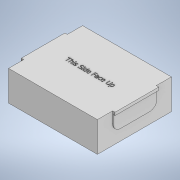
# Autodesk Inventor part: iRobot_filter
Saved by Autodesk Inventor 2020 (Build 240168000, 168)
## iProperties
Created: 2020-04-05
Part Number: iRobot_filter
Material: Generic
Document SubType Name: Modeling
Designer: Clevo
Density: 1 g/cm^3
Appearance: Default
Author: Clevo
Autodesk Inventor part; units mm, degrees
ref_plane "YZ Plane" through (0, 0, 0) normal (1, 0, 0) x (0, 1, 0)
ref_plane "XZ Plane" through (0, 0, 0) normal (0, 1, 0) x (-1, 0, 0)
ref_plane "XY Plane" through (0, 0, 0) normal (0, 0, 1) x (1, 0, 0)
sketch "Sketch1" plane through (0, 0, 0) normal (0, 1, 0) x (-1, 0, 0)
  line L0 (-30.48, -25.4) -> (30.48, -25.4)
  line L1 (30.48, -25.4) -> (30.48, 25.4)
  line L2 (30.48, 25.4) -> (-30.48, 25.4)
  line L3 (-30.48, 25.4) -> (-30.48, -25.4)
  line L4 (-30.48, -25.4) -> (30.48, 25.4) construction
  line L5 (30.48, -25.4) -> (-30.48, 25.4) construction
  point P0 (0, 0)
  dimension "d0" = 50.8
  dimension "d1" = 60.96
  constraints: 12 end point, 2 midpoint, 2 parallel, 1 horizontal, 1 perpendicular
  measures "d0" distance of L0.end L1.end
  measures "d1" distance of L1.end L2.end
extrude "Extrusion1" add sketch "Sketch1" along normal blind 20.6629
sketch "Sketch2" plane through (30.48, 0, 25.4) normal (1, 0, 0) x (0, 0, -1)
  line L0 (0, 0) -> (50.8, 0) projected
  line L1 (50.8, 0) -> (50.8, 20.6629) projected
  line L2 (0, 20.6629) -> (50.8, 20.6629) projected
  line L3 (0, 0) -> (0, 20.6629) projected
  line L4 (0, 20.6629) -> (50.8, 20.6629) projected
  line L5 (10.4, 20.6629) -> (40.4, 20.6629)
  line L6 (40.4, 20.6629) -> (40.4, 7.9629)
  line L7 (40.4, 7.9629) -> (10.4, 7.9629)
  line L8 (10.4, 7.9629) -> (10.4, 20.6629)
  point P0 (25.4, 0)
  point P1 (25.4, 20.6629)
  point P2 (25.4, 20.6629)
  point P3 (10.4, 20.6629)
  dimension "d4" = 12.7
  dimension "d5" = 30
  constraints: 8 end point, 2 midpoint, 2 parallel, 1 coincident, 1 horizontal, 1 perpendicular, 1 point on line
  measures "d4" distance of L5.end L6.end
  measures "d5" distance of L6.end L7.end
extrude "Extrusion2" add sketch "Sketch2" along normal blind 0.5 contours L2 L6 L7 L8
fillet "Fillet1" radius 5 2 edges at (30.73, 7.9629, 15) (30.73, 7.9629, -15)
sketch "Sketch3" plane through (30.98, 0, 25.4) normal (1, 0, 0) x (0, 0, -1)
  arc A0 (35.4, 7.9629) -> (40.4, 12.9629) centre (35.4, 12.9629) ccw projected
  line L0 (40.4, 12.9629) -> (40.4, 20.6629) projected
  line L1 (40.4, 20.6629) -> (10.4, 20.6629) projected
  line L2 (10.4, 20.6629) -> (10.4, 12.9629) projected
  arc A1 (10.4, 12.9629) -> (15.4, 7.9629) centre (15.4, 12.9629) ccw projected
  line L3 (15.4, 7.9629) -> (35.4, 7.9629) projected
  line L4 (40.4, 20.6629) -> (10.4, 20.6629) projected
  line L5 (40.4, 12.9629) -> (40.4, 20.6629) projected
  line L6 (10.4, 20.6629) -> (40.4, 20.6629)
  line L7 (40.4, 20.6629) -> (40.4, 18.6629)
  line L8 (40.4, 18.6629) -> (10.4, 18.6629)
  line L9 (10.4, 18.6629) -> (10.4, 20.6629)
  point P0 (25.4, 0)
  point P1 (10.4, 18.6629)
  dimension "d9" = 2
  constraints: 8 end point, 2 parallel, 1 horizontal, 1 perpendicular, 1 point on line
  measures "d9" distance between parallel lines of L1 L8
extrude "Extrusion3" add sketch "Sketch3" along normal blind 1.17 contours L8 L2 L1 L0
mirror "Mirror1" about plane through (0, 0, 0) normal (1, 0, 0) of "Extrusion2", "Fillet1", "Extrusion3"
sketch "Sketch4" plane through (0, 20.6629, 0) normal (0, 1, 0) x (1, 0, 0)
  line L0 (-16.5843, 2.036) -> (16.3633, 2.036) construction
  line L1 (16.3633, 2.036) -> (16.3633, -1.9901) construction
  line L2 (16.3633, -1.9901) -> (-16.5843, -1.9901) construction
  line L3 (-16.5843, -1.9901) -> (-16.5843, 2.036) construction
  line L4 (-15.5642, -1.1479) -> (-15.5642, 1.5395)
  line L5 (-15.5642, 1.5395) -> (-16.5867, 1.5395)
  line L6 (-16.5867, 1.5395) -> (-16.5867, 1.9001)
  line L7 (-16.5867, 1.9001) -> (-14.1365, 1.9001)
  line L8 (-14.1365, 1.9001) -> (-14.1365, 1.5395)
  line L9 (-14.1365, 1.5395) -> (-15.1591, 1.5395)
  line L10 (-15.1591, 1.5395) -> (-15.1591, -1.1479)
  line L11 (-15.1591, -1.1479) -> (-15.5642, -1.1479)
  line L12 (-12.0617, -1.1479) -> (-12.447, -1.1479)
  line L13 (-12.447, -1.1479) -> (-12.447, 0.1563)
  spline S0 degree 2 poles (-12.447, 0.1563) (-12.447, 0.3144) (-12.4766, 0.5861) (-12.5211, 0.6676) knots 0 0 0 1 2 2 2
  spline S1 degree 2 poles (-12.5211, 0.6676) (-12.568, 0.7541) (-12.736, 0.838) (-12.8792, 0.838) knots 0 0 0 1 2 2 2
  spline S2 degree 2 poles (-12.8792, 0.838) (-13.0225, 0.838) (-13.3263, 0.6849) (-13.472, 0.5614) knots 0 0 0 1 2 2 2
  line L14 (-13.472, 0.5614) -> (-13.472, -1.1479)
  line L15 (-13.472, -1.1479) -> (-13.8574, -1.1479)
  line L16 (-13.8574, -1.1479) -> (-13.8574, 2.036)
  line L17 (-13.8574, 2.036) -> (-13.472, 2.036)
  line L18 (-13.472, 2.036) -> (-13.472, 0.885)
  spline S3 degree 2 poles (-13.472, 0.885) (-13.2991, 1.0406) (-12.9657, 1.2036) (-12.778, 1.2036) knots 0 0 0 1 2 2 2
  spline S4 degree 2 poles (-12.778, 1.2036) (-12.4421, 1.2036) (-12.0617, 0.759) (-12.0617, 0.3366) knots 0 0 0 1 2 2 2
  line L19 (-12.0617, 0.3366) -> (-12.0617, -1.1479)
  line L20 (-11.128, -1.1479) -> (-11.5133, -1.1479)
  line L21 (-11.5133, -1.1479) -> (-11.5133, 1.1394)
  line L22 (-11.5133, 1.1394) -> (-11.128, 1.1394)
  line L23 (-11.128, 1.1394) -> (-11.128, -1.1479)
  line L24 (-11.1008, 1.5198) -> (-11.538, 1.5198)
  line L25 (-11.538, 1.5198) -> (-11.538, 1.9199)
  line L26 (-11.538, 1.9199) -> (-11.1008, 1.9199)
  line L27 (-11.1008, 1.9199) -> (-11.1008, 1.5198)
  spline S5 degree 2 poles (-9.9449, -1.2022) (-10.1746, -1.2022) (-10.5722, -1.0787) (-10.7032, -1.0095) knots 0 0 0 1 2 2 2
  line L28 (-10.7032, -1.0095) -> (-10.7032, -0.5773)
  line L29 (-10.7032, -0.5773) -> (-10.6834, -0.5773)
  spline S6 degree 2 poles (-10.6834, -0.5773) (-10.634, -0.6168) (-10.5006, -0.7107) (-10.3895, -0.7625) knots 0 0 0 1 2 2 2
  spline S7 degree 2 poles (-10.3895, -0.7625) (-10.2931, -0.8095) (-10.056, -0.8786) (-9.93, -0.8786) knots 0 0 0 1 2 2 2
  spline S8 degree 2 poles (-9.93, -0.8786) (-9.8387, -0.8786) (-9.6287, -0.8366) (-9.5793, -0.8021) knots 0 0 0 1 2 2 2
  spline S9 degree 2 poles (-9.5793, -0.8021) (-9.5077, -0.7551) (-9.4435, -0.6489) (-9.4435, -0.5402) knots 0 0 0 1 2 2 2
  spline S10 degree 2 poles (-9.4435, -0.5402) (-9.4435, -0.4044) (-9.5917, -0.2636) (-9.7818, -0.2167) knots 0 0 0 1 2 2 2
  spline S11 degree 2 poles (-9.7818, -0.2167) (-9.8559, -0.1994) (-10.0931, -0.15) (-10.1943, -0.1228) knots 0 0 0 1 2 2 2
  spline S12 degree 2 poles (-10.1943, -0.1228) (-10.4562, -0.0462) (-10.6933, 0.2699) (-10.6933, 0.4947) knots 0 0 0 1 2 2 2
  spline S13 degree 2 poles (-10.6933, 0.4947) (-10.6933, 0.8059) (-10.2264, 1.1937) (-9.8411, 1.1937) knots 0 0 0 1 2 2 2
  spline S14 degree 2 poles (-9.8411, 1.1937) (-9.6509, 1.1937) (-9.2656, 1.0999) (-9.1347, 1.0282) knots 0 0 0 1 2 2 2
  line L30 (-9.1347, 1.0282) -> (-9.1347, 0.6157)
  line L31 (-9.1347, 0.6157) -> (-9.1545, 0.6157)
  spline S15 degree 2 poles (-9.1545, 0.6157) (-9.3027, 0.7343) (-9.6633, 0.8701) (-9.8485, 0.8701) knots 0 0 0 1 2 2 2
  spline S16 degree 2 poles (-9.8485, 0.8701) (-10.0387, 0.8701) (-10.3005, 0.7096) (-10.3005, 0.549) knots 0 0 0 1 2 2 2
  spline S17 degree 2 poles (-10.3005, 0.549) (-10.3005, 0.4033) (-10.1449, 0.2625) (-9.972, 0.2181) knots 0 0 0 1 2 2 2
  spline S18 degree 2 poles (-9.972, 0.2181) (-9.8881, 0.1958) (-9.6756, 0.1514) (-9.5595, 0.1242) knots 0 0 0 1 2 2 2
  spline S19 degree 2 poles (-9.5595, 0.1242) (-9.3076, 0.06) (-9.0507, -0.2339) (-9.0507, -0.4884) knots 0 0 0 1 2 2 2
  spline S20 degree 2 poles (-9.0507, -0.4884) (-9.0507, -0.6366) (-9.1668, -0.8984) (-9.2804, -0.9947) knots 0 0 0 1 2 2 2
  spline S21 degree 2 poles (-9.2804, -0.9947) (-9.4015, -1.096) (-9.7102, -1.2022) (-9.9449, -1.2022) knots 0 0 0 1 2 2 2
  spline S22 degree 2 poles (-6.5041, -1.2022) (-6.8351, -1.2022) (-7.2995, -1.0639) (-7.5045, -0.9651) knots 0 0 0 1 2 2 2
  line L32 (-7.5045, -0.9651) -> (-7.5045, -0.4563)
  line L33 (-7.5045, -0.4563) -> (-7.4748, -0.4563)
  spline S23 degree 2 poles (-7.4748, -0.4563) (-7.2748, -0.644) (-6.7684, -0.8515) (-6.5338, -0.8515) knots 0 0 0 1 2 2 2
  spline S24 degree 2 poles (-6.5338, -0.8515) (-6.1978, -0.8515) (-5.8545, -0.5723) (-5.8545, -0.3426) knots 0 0 0 1 2 2 2
  spline S25 degree 2 poles (-5.8545, -0.3426) (-5.8545, -0.1598) (-6.0348, 0.0674) (-6.23, 0.1242) knots 0 0 0 1 2 2 2
  spline S26 degree 2 poles (-6.23, 0.1242) (-6.3708, 0.1637) (-6.6054, 0.2181) (-6.7808, 0.2625) knots 0 0 0 1 2 2 2
  spline S27 degree 2 poles (-6.7808, 0.2625) (-6.9389, 0.3045) (-7.1883, 0.4305) (-7.2847, 0.5318) knots 0 0 0 1 2 2 2
  spline S28 degree 2 poles (-7.2847, 0.5318) (-7.3785, 0.633) (-7.4823, 0.9047) (-7.4823, 1.0826) knots 0 0 0 1 2 2 2
  spline S29 degree 2 poles (-7.4823, 1.0826) (-7.4823, 1.4531) (-6.9043, 1.9545) (-6.4572, 1.9545) knots 0 0 0 1 2 2 2
  spline S30 degree 2 poles (-6.4572, 1.9545) (-6.2003, 1.9545) (-5.7458, 1.8532) (-5.5507, 1.7569) knots 0 0 0 1 2 2 2
  line L34 (-5.5507, 1.7569) -> (-5.5507, 1.2728)
  line L35 (-5.5507, 1.2728) -> (-5.5803, 1.2728)
  spline S31 degree 2 poles (-5.5803, 1.2728) (-5.7261, 1.4061) (-6.1806, 1.6037) (-6.43, 1.6037) knots 0 0 0 1 2 2 2
  spline S32 degree 2 poles (-6.43, 1.6037) (-6.7116, 1.6037) (-7.0599, 1.3395) (-7.0599, 1.1246) knots 0 0 0 1 2 2 2
  spline S33 degree 2 poles (-7.0599, 1.1246) (-7.0599, 0.9319) (-6.8549, 0.7022) (-6.6622, 0.6503) knots 0 0 0 1 2 2 2
  spline S34 degree 2 poles (-6.6622, 0.6503) (-6.5338, 0.6157) (-6.1608, 0.5268) (-6.0373, 0.4898) knots 0 0 0 1 2 2 2
  spline S35 degree 2 poles (-6.0373, 0.4898) (-5.7236, 0.3934) (-5.4321, 0.0056) (-5.4321, -0.2784) knots 0 0 0 1 2 2 2
  spline S36 degree 2 poles (-5.4321, -0.2784) (-5.4321, -0.4587) (-5.5779, -0.8045) (-5.7088, -0.9256) knots 0 0 0 1 2 2 2
  spline S37 degree 2 poles (-5.7088, -0.9256) (-5.8545, -1.0589) (-6.225, -1.2022) (-6.5041, -1.2022) knots 0 0 0 1 2 2 2
  line L36 (-4.6566, -1.1479) -> (-5.0419, -1.1479)
  line L37 (-5.0419, -1.1479) -> (-5.0419, 1.1394)
  line L38 (-5.0419, 1.1394) -> (-4.6566, 1.1394)
  line L39 (-4.6566, 1.1394) -> (-4.6566, -1.1479)
  line L40 (-4.6294, 1.5198) -> (-5.0666, 1.5198)
  line L41 (-5.0666, 1.5198) -> (-5.0666, 1.9199)
  line L42 (-5.0666, 1.9199) -> (-4.6294, 1.9199)
  line L43 (-4.6294, 1.9199) -> (-4.6294, 1.5198)
  line L44 (-2.3323, -1.1479) -> (-2.7176, -1.1479)
  line L45 (-2.7176, -1.1479) -> (-2.7176, -0.9157)
  spline S38 degree 2 poles (-2.7176, -0.9157) (-2.8065, -0.9898) (-2.9374, -1.0886) (-3.0263, -1.1306) knots 0 0 0 1 2 2 2
  spline S39 degree 2 poles (-3.0263, -1.1306) (-3.1079, -1.1701) (-3.2832, -1.2121) (-3.3993, -1.2121) knots 0 0 0 1 2 2 2
  spline S40 degree 2 poles (-3.3993, -1.2121) (-3.587, -1.2121) (-3.9032, -1.0565) (-4.0144, -0.9058) knots 0 0 0 1 2 2 2
  spline S41 degree 2 poles (-4.0144, -0.9058) (-4.1255, -0.7551) (-4.249, -0.3105) (-4.249, -0.0215) knots 0 0 0 1 2 2 2
  spline S42 degree 2 poles (-4.249, -0.0215) (-4.249, 0.2798) (-4.0934, 0.7195) (-3.9575, 0.885) knots 0 0 0 1 2 2 2
  spline S43 degree 2 poles (-3.9575, 0.885) (-3.8316, 1.0332) (-3.4784, 1.2036) (-3.2832, 1.2036) knots 0 0 0 1 2 2 2
  spline S44 degree 2 poles (-3.2832, 1.2036) (-3.1128, 1.2036) (-2.8584, 1.127) (-2.7176, 1.048) knots 0 0 0 1 2 2 2
  line L46 (-2.7176, 1.048) -> (-2.7176, 2.036)
  line L47 (-2.7176, 2.036) -> (-2.3323, 2.036)
  line L48 (-2.3323, 2.036) -> (-2.3323, -1.1479)
  line L49 (-2.7176, -0.5921) -> (-2.7176, 0.7294)
  spline S45 degree 2 poles (-2.7176, 0.7294) (-2.8609, 0.7985) (-3.0881, 0.8504) (-3.219, 0.8504) knots 0 0 0 1 2 2 2
  spline S46 degree 2 poles (-3.219, 0.8504) (-3.5154, 0.8504) (-3.8513, 0.4058) (-3.8513, -0.0141) knots 0 0 0 1 2 2 2
  spline S47 degree 2 poles (-3.8513, -0.0141) (-3.8513, -0.4192) (-3.5945, -0.8465) (-3.3104, -0.8465) knots 0 0 0 1 2 2 2
  spline S48 degree 2 poles (-3.3104, -0.8465) (-3.1597, -0.8465) (-2.8534, -0.7082) (-2.7176, -0.5921) knots 0 0 0 1 2 2 2
  spline S49 degree 2 poles (-0.7811, -1.1997) (-1.3294, -1.1997) (-1.9321, -0.5847) (-1.9321, -0.0166) knots 0 0 0 1 2 2 2
  spline S50 degree 2 poles (-1.9321, -0.0166) (-1.9321, 0.5416) (-1.3467, 1.2036) (-0.875, 1.2036) knots 0 0 0 1 2 2 2
  spline S51 degree 2 poles (-0.875, 1.2036) (-0.6625, 1.2036) (-0.334, 1.0801) (-0.213, 0.9492) knots 0 0 0 1 2 2 2
  spline S52 degree 2 poles (-0.213, 0.9492) (-0.0895, 0.8183) (0.0414, 0.4404) (0.0414, 0.1662) knots 0 0 0 1 2 2 2
  line L50 (0.0414, 0.1662) -> (0.0414, -0.0438)
  line L51 (0.0414, -0.0438) -> (-1.5419, -0.0438)
  spline S53 degree 2 poles (-1.5419, -0.0438) (-1.5419, -0.4414) (-1.1417, -0.8638) (-0.786, -0.8638) knots 0 0 0 1 2 2 2
  spline S54 degree 2 poles (-0.786, -0.8638) (-0.6601, -0.8638) (-0.4155, -0.807) (-0.3167, -0.7625) knots 0 0 0 1 2 2 2
  spline S55 degree 2 poles (-0.3167, -0.7625) (-0.213, -0.7131) (-0.0697, -0.6267) (-0.0228, -0.5872) knots 0 0 0 1 2 2 2
  line L52 (-0.0228, -0.5872) -> (-0.0006, -0.5872)
  line L53 (-0.0006, -0.5872) -> (-0.0006, -1.0071)
  spline S56 degree 2 poles (-0.0006, -1.0071) (-0.0673, -1.0342) (-0.2698, -1.1133) (-0.3489, -1.1355) knots 0 0 0 1 2 2 2
  spline S57 degree 2 poles (-0.3489, -1.1355) (-0.46, -1.1676) (-0.6428, -1.1997) (-0.7811, -1.1997) knots 0 0 0 1 2 2 2
  spline S58 degree 2 poles (-0.334, 0.2502) (-0.339, 0.4058) (-0.4032, 0.633) (-0.4649, 0.7096) knots 0 0 0 1 2 2 2
  spline S59 degree 2 poles (-0.4649, 0.7096) (-0.5316, 0.796) (-0.7416, 0.8874) (-0.8972, 0.8874) knots 0 0 0 1 2 2 2
  spline S60 degree 2 poles (-0.8972, 0.8874) (-1.0503, 0.8874) (-1.2652, 0.796) (-1.3541, 0.7071) knots 0 0 0 1 2 2 2
  spline S61 degree 2 poles (-1.3541, 0.7071) (-1.4406, 0.6157) (-1.5295, 0.3959) (-1.5419, 0.2502) knots 0 0 0 1 2 2 2
  line L54 (-1.5419, 0.2502) -> (-0.334, 0.2502)
  line L55 (3.5933, 1.5395) -> (2.1755, 1.5395)
  line L56 (2.1755, 1.5395) -> (2.1755, 0.68)
  line L57 (2.1755, 0.68) -> (3.534, 0.68)
  line L58 (3.534, 0.68) -> (3.534, 0.3193)
  line L59 (3.534, 0.3193) -> (2.1755, 0.3193)
  line L60 (2.1755, 0.3193) -> (2.1755, -1.1479)
  line L61 (2.1755, -1.1479) -> (1.7704, -1.1479)
  line L62 (1.7704, -1.1479) -> (1.7704, 1.9001)
  line L63 (1.7704, 1.9001) -> (3.5933, 1.9001)
  line L64 (3.5933, 1.9001) -> (3.5933, 1.5395)
  spline S62 degree 2 poles (5.2013, -0.9058) (5.1543, -0.9404) (4.9963, -1.0639) (4.9222, -1.1009) knots 0 0 0 1 2 2 2
  spline S63 degree 2 poles (4.9222, -1.1009) (4.8209, -1.1553) (4.6307, -1.2121) (4.4578, -1.2121) knots 0 0 0 1 2 2 2
  spline S64 degree 2 poles (4.4578, -1.2121) (4.317, -1.2121) (4.0626, -1.1059) (3.9663, -1.0095) knots 0 0 0 1 2 2 2
  spline S65 degree 2 poles (3.9663, -1.0095) (3.8749, -0.9157) (3.7637, -0.639) (3.7637, -0.4859) knots 0 0 0 1 2 2 2
  spline S66 degree 2 poles (3.7637, -0.4859) (3.7637, -0.2488) (3.9638, 0.0872) (4.1812, 0.1835) knots 0 0 0 1 2 2 2
  spline S67 degree 2 poles (4.1812, 0.1835) (4.3738, 0.2724) (4.8975, 0.3391) (5.2013, 0.3564) knots 0 0 0 1 2 2 2
  line L65 (5.2013, 0.3564) -> (5.2013, 0.4305)
  spline S68 degree 2 poles (5.2013, 0.4305) (5.2013, 0.5639) (5.1198, 0.7294) (5.0457, 0.7763) knots 0 0 0 1 2 2 2
  spline S69 degree 2 poles (5.0457, 0.7763) (4.9716, 0.8232) (4.7591, 0.8529) (4.6455, 0.8529) knots 0 0 0 1 2 2 2
  spline S70 degree 2 poles (4.6455, 0.8529) (4.5121, 0.8529) (4.1515, 0.7738) (3.9712, 0.6972) knots 0 0 0 1 2 2 2
  line L66 (3.9712, 0.6972) -> (3.949, 0.6972)
  line L67 (3.949, 0.6972) -> (3.949, 1.09)
  spline S71 degree 2 poles (3.949, 1.09) (4.0552, 1.1196) (4.4529, 1.1937) (4.648, 1.1937) knots 0 0 0 1 2 2 2
  spline S72 degree 2 poles (4.648, 1.1937) (4.8851, 1.1937) (5.2087, 1.1196) (5.3371, 1.0233) knots 0 0 0 1 2 2 2
  spline S73 degree 2 poles (5.3371, 1.0233) (5.4631, 0.9294) (5.5866, 0.6306) (5.5866, 0.4157) knots 0 0 0 1 2 2 2
  line L68 (5.5866, 0.4157) -> (5.5866, -1.1479)
  line L69 (5.5866, -1.1479) -> (5.2013, -1.1479)
  line L70 (5.2013, -1.1479) -> (5.2013, -0.9058)
  line L71 (5.2013, -0.5847) -> (5.2013, 0.0501)
  spline S74 degree 2 poles (5.2013, 0.0501) (5.063, 0.0378) (4.6455, -0.0042) (4.5146, -0.0438) knots 0 0 0 1 2 2 2
  spline S75 degree 2 poles (4.5146, -0.0438) (4.3615, -0.0907) (4.1614, -0.2858) (4.1614, -0.4587) knots 0 0 0 1 2 2 2
  spline S76 degree 2 poles (4.1614, -0.4587) (4.1614, -0.6563) (4.3837, -0.8564) (4.5961, -0.8564) knots 0 0 0 1 2 2 2
  spline S77 degree 2 poles (4.5961, -0.8564) (4.7764, -0.8564) (5.0728, -0.7008) (5.2013, -0.5847) knots 0 0 0 1 2 2 2
  spline S78 degree 2 poles (7.0365, -1.1997) (6.7994, -1.1997) (6.4066, -1.054) (6.2659, -0.9058) knots 0 0 0 1 2 2 2
  spline S79 degree 2 poles (6.2659, -0.9058) (6.1251, -0.7601) (5.9695, -0.3105) (5.9695, -0.0092) knots 0 0 0 1 2 2 2
  spline S80 degree 2 poles (5.9695, -0.0092) (5.9695, 0.2922) (6.13, 0.7318) (6.2659, 0.88) knots 0 0 0 1 2 2 2
  spline S81 degree 2 poles (6.2659, 0.88) (6.4017, 1.0307) (6.8043, 1.1913) (7.0365, 1.1913) knots 0 0 0 1 2 2 2
  spline S82 degree 2 poles (7.0365, 1.1913) (7.2242, 1.1913) (7.575, 1.085) (7.7108, 1.0159) knots 0 0 0 1 2 2 2
  line L72 (7.7108, 1.0159) -> (7.7108, 0.5836)
  line L73 (7.7108, 0.5836) -> (7.6886, 0.5836)
  spline S83 degree 2 poles (7.6886, 0.5836) (7.6466, 0.6182) (7.5182, 0.7071) (7.4268, 0.7541) knots 0 0 0 1 2 2 2
  spline S84 degree 2 poles (7.4268, 0.7541) (7.3452, 0.7936) (7.1279, 0.8553) (7.0291, 0.8553) knots 0 0 0 1 2 2 2
  spline S85 degree 2 poles (7.0291, 0.8553) (6.7302, 0.8553) (6.3671, 0.4033) (6.3671, -0.0092) knots 0 0 0 1 2 2 2
  spline S86 degree 2 poles (6.3671, -0.0092) (6.3671, -0.4118) (6.7179, -0.8638) (7.0291, -0.8638) knots 0 0 0 1 2 2 2
  spline S87 degree 2 poles (7.0291, -0.8638) (7.2168, -0.8638) (7.5577, -0.7082) (7.6886, -0.5872) knots 0 0 0 1 2 2 2
  line L74 (7.6886, -0.5872) -> (7.7108, -0.5872)
  line L75 (7.7108, -0.5872) -> (7.7108, -1.0194)
  spline S88 degree 2 poles (7.7108, -1.0194) (7.654, -1.0466) (7.4811, -1.1232) (7.4119, -1.1404) knots 0 0 0 1 2 2 2
  spline S89 degree 2 poles (7.4119, -1.1404) (7.3131, -1.1701) (7.1575, -1.1997) (7.0365, -1.1997) knots 0 0 0 1 2 2 2
  spline S90 degree 2 poles (9.0545, -1.1997) (8.5062, -1.1997) (7.9035, -0.5847) (7.9035, -0.0166) knots 0 0 0 1 2 2 2
  spline S91 degree 2 poles (7.9035, -0.0166) (7.9035, 0.5416) (8.4889, 1.2036) (8.9606, 1.2036) knots 0 0 0 1 2 2 2
  spline S92 degree 2 poles (8.9606, 1.2036) (9.1731, 1.2036) (9.5016, 1.0801) (9.6226, 0.9492) knots 0 0 0 1 2 2 2
  spline S93 degree 2 poles (9.6226, 0.9492) (9.7461, 0.8183) (9.877, 0.4404) (9.877, 0.1662) knots 0 0 0 1 2 2 2
  line L76 (9.877, 0.1662) -> (9.877, -0.0438)
  line L77 (9.877, -0.0438) -> (8.2937, -0.0438)
  spline S94 degree 2 poles (8.2937, -0.0438) (8.2937, -0.4414) (8.6939, -0.8638) (9.0496, -0.8638) knots 0 0 0 1 2 2 2
  spline S95 degree 2 poles (9.0496, -0.8638) (9.1755, -0.8638) (9.4201, -0.807) (9.5189, -0.7625) knots 0 0 0 1 2 2 2
  spline S96 degree 2 poles (9.5189, -0.7625) (9.6226, -0.7131) (9.7659, -0.6267) (9.8128, -0.5872) knots 0 0 0 1 2 2 2
  line L78 (9.8128, -0.5872) -> (9.835, -0.5872)
  line L79 (9.835, -0.5872) -> (9.835, -1.0071)
  spline S97 degree 2 poles (9.835, -1.0071) (9.7683, -1.0342) (9.5658, -1.1133) (9.4868, -1.1355) knots 0 0 0 1 2 2 2
  spline S98 degree 2 poles (9.4868, -1.1355) (9.3756, -1.1676) (9.1928, -1.1997) (9.0545, -1.1997) knots 0 0 0 1 2 2 2
  spline S99 degree 2 poles (9.5016, 0.2502) (9.4966, 0.4058) (9.4324, 0.633) (9.3707, 0.7096) knots 0 0 0 1 2 2 2
  spline S100 degree 2 poles (9.3707, 0.7096) (9.304, 0.796) (9.094, 0.8874) (8.9384, 0.8874) knots 0 0 0 1 2 2 2
  spline S101 degree 2 poles (8.9384, 0.8874) (8.7853, 0.8874) (8.5704, 0.796) (8.4815, 0.7071) knots 0 0 0 1 2 2 2
  spline S102 degree 2 poles (8.4815, 0.7071) (8.395, 0.6157) (8.3061, 0.3959) (8.2937, 0.2502) knots 0 0 0 1 2 2 2
  line L80 (8.2937, 0.2502) -> (9.5016, 0.2502)
  spline S103 degree 2 poles (12.6706, -1.2121) (12.4014, -1.2121) (12.0012, -1.0713) (11.8604, -0.9305) knots 0 0 0 1 2 2 2
  spline S104 degree 2 poles (11.8604, -0.9305) (11.6999, -0.7724) (11.569, -0.3278) (11.569, -0.0018) knots 0 0 0 1 2 2 2
  line L81 (11.569, -0.0018) -> (11.569, 1.9001)
  line L82 (11.569, 1.9001) -> (11.9741, 1.9001)
  line L83 (11.9741, 1.9001) -> (11.9741, -0.0018)
  spline S105 degree 2 poles (11.9741, -0.0018) (11.9741, -0.2142) (12.0284, -0.5007) (12.105, -0.6168) knots 0 0 0 1 2 2 2
  spline S106 degree 2 poles (12.105, -0.6168) (12.1865, -0.7403) (12.4681, -0.8663) (12.6706, -0.8663) knots 0 0 0 1 2 2 2
  spline S107 degree 2 poles (12.6706, -0.8663) (12.8608, -0.8663) (13.1572, -0.7403) (13.2387, -0.6168) knots 0 0 0 1 2 2 2
  spline S108 degree 2 poles (13.2387, -0.6168) (13.3153, -0.5007) (13.3696, -0.2167) (13.3696, -0.0116) knots 0 0 0 1 2 2 2
  line L84 (13.3696, -0.0116) -> (13.3696, 1.9001)
  line L85 (13.3696, 1.9001) -> (13.7747, 1.9001)
  line L86 (13.7747, 1.9001) -> (13.7747, -0.0018)
  spline S109 degree 2 poles (13.7747, -0.0018) (13.7747, -0.3204) (13.6463, -0.7749) (13.4832, -0.9305) knots 0 0 0 1 2 2 2
  spline S110 degree 2 poles (13.4832, -0.9305) (13.3375, -1.0738) (12.9522, -1.2121) (12.6706, -1.2121) knots 0 0 0 1 2 2 2
  spline S111 degree 2 poles (16.2422, 0.0575) (16.2422, -0.5155) (15.6964, -1.1923) (15.2789, -1.1923) knots 0 0 0 1 2 2 2
  spline S112 degree 2 poles (15.2789, -1.1923) (15.1085, -1.1923) (14.8467, -1.1133) (14.7108, -1.0318) knots 0 0 0 1 2 2 2
  line L87 (14.7108, -1.0318) -> (14.7108, -1.9901)
  line L88 (14.7108, -1.9901) -> (14.3255, -1.9901)
  line L89 (14.3255, -1.9901) -> (14.3255, 1.1394)
  line L90 (14.3255, 1.1394) -> (14.7108, 1.1394)
  line L91 (14.7108, 1.1394) -> (14.7108, 0.8998)
  spline S113 degree 2 poles (14.7108, 0.8998) (14.8541, 1.0307) (15.2048, 1.2036) (15.4099, 1.2036) knots 0 0 0 1 2 2 2
  spline S114 degree 2 poles (15.4099, 1.2036) (15.8026, 1.2036) (16.2422, 0.5812) (16.2422, 0.0575) knots 0 0 0 1 2 2 2
  spline S115 degree 2 poles (15.8446, 0.0131) (15.8446, 0.4058) (15.5951, 0.838) (15.316, 0.838) knots 0 0 0 1 2 2 2
  spline S116 degree 2 poles (15.316, 0.838) (15.153, 0.838) (14.8467, 0.6923) (14.7108, 0.5787) knots 0 0 0 1 2 2 2
  line L92 (14.7108, 0.5787) -> (14.7108, -0.7205)
  spline S117 degree 2 poles (14.7108, -0.7205) (14.8615, -0.7922) (15.0764, -0.8465) (15.2147, -0.8465) knots 0 0 0 1 2 2 2
  spline S118 degree 2 poles (15.2147, -0.8465) (15.5136, -0.8465) (15.8446, -0.4068) (15.8446, 0.0131) knots 0 0 0 1 2 2 2
  point P0 (0, 0)
  constraints: 2 other
extrude "Extrusion4" cut sketch "Sketch4" against normal blind 1
body "Solid1"
